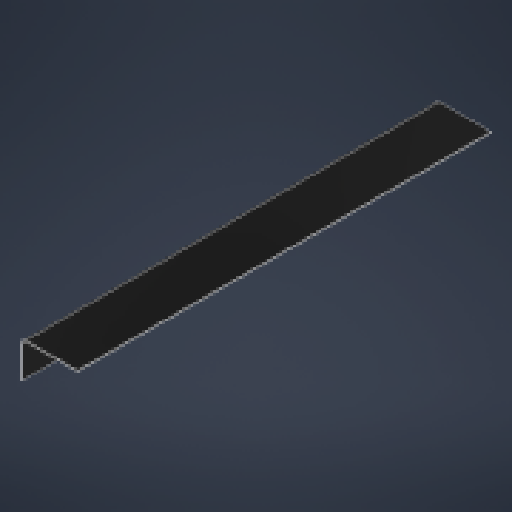
# Autodesk Inventor part: TopPlate
Saved by Autodesk Inventor 2023 (Build 270158000, 158)
## iProperties
Created: 2022-11-17
Part Number: TopPlate
Material: ABS Plastic
Document SubType Name: Modeling
Designer: kumpu
Density: 1.06 g/cm^3
Appearance: Smooth - Black
Mass: 160.66 g
Surface Area: 1935.06 cm^2
Volume: 151.566 cm^3
Author: kumpu
Autodesk Inventor part; units mm, degrees
ref_plane "YZ Plane" through (0, 0, 0) normal (1, 0, 0) x (0, 1, 0)
ref_plane "XZ Plane" through (0, 0, 0) normal (0, 1, 0) x (-1, 0, 0)
ref_plane "XY Plane" through (0, 0, 0) normal (0, 0, 1) x (1, 0, 0)
sketch "Sketch1" plane through (0, 0, 0) normal (0, 1, 0) x (-1, 0, 0)
  line L0 (41.275, 330.2) -> (-41.275, 330.2)
  line L1 (-41.275, 330.2) -> (-41.275, -330.2)
  line L2 (-41.275, -330.2) -> (41.275, -330.2)
  line L3 (41.275, -330.2) -> (41.275, 330.2)
  line L4 (41.275, 330.2) -> (-41.275, -330.2) construction
  line L5 (-41.275, 330.2) -> (41.275, -330.2) construction
  point P0 (0, 0)
  dimension "d0" = 82.55
  dimension "d1" = 660.4
  constraints: 12 end point, 2 midpoint, 2 parallel, 1 horizontal, 1 perpendicular
  measures "d0" distance of L2.end L1.end
  measures "d1" distance of L1.end L0.end
extrude "Extrusion1" add sketch "Sketch1" along normal mid plane 1.5875
sketch "Sketch2" plane through (41.275, 0.7937, -330.2) normal (0, 0, -1) x (-1, 0, 0)
  line L0 (90.4875, -7.9375) -> (90.4875, -58.7375)
  line L1 (90.4875, -58.7375) -> (88.9, -58.7375)
  line L2 (88.9, -58.7375) -> (88.9, -7.9375)
  arc A0 (88.9, -7.9375) -> (82.55, -1.5875) centre (82.55, -7.9375) ccw
  line L3 (82.55, -1.5875) -> (82.55, 0)
  arc A1 (90.4875, -7.9375) -> (82.55, 0) centre (82.55, -7.9375) ccw
  point P0 (41.275, -0.7937)
  dimension "d4" = 6.35
  dimension "d5" = 57.15
  dimension "d6" = 1.5875
  constraints: 8 end point, 4 point on circle, 2 centre point, 2 line through centre, 2 perpendicular, 2 tangent, 1 coincident, 1 concentric, 1 parallel, 1 point on line, 1 vertical
  measures "d4" radius of A0
  measures "d5" distance from line of L1 L3.start
  measures "d6" distance of L3.start L3.end
extrude "Extrusion2" add sketch "Sketch2" against normal blind 660.4
sketch "Sketch3" plane through (-49.2125, -57.9438, -330.2) normal (-1, 0, 0) x (0, 0, 1)
  arc A0 (518.9985, 0) -> (520.5697, 1.8143) centre (518.9985, 1.5875) ccw projected
  arc A1 (520.5697, 1.8143) -> (508, 12.7) centre (508, 0) ccw projected
  line L0 (497.2617, 12.7) -> (508, 12.7) projected
  line L1 (413.9219, 12.7) -> (497.2617, 12.7) projected
  line L2 (330.2, 12.7) -> (413.9219, 12.7) projected
  line L3 (226.8601, 12.7) -> (330.2, 12.7) projected
  line L4 (158.6559, 12.7) -> (226.8601, 12.7) projected
  line L5 (152.4, 12.7) -> (158.6559, 12.7) projected
  arc A2 (152.4, 12.7) -> (139.8303, 1.8143) centre (152.4, 0) ccw projected
  arc A3 (139.8303, 1.8143) -> (141.4015, 0) centre (141.4015, 1.5875) ccw projected
  line L6 (518.9985, 0) -> (141.4015, 0) projected
  line L7 (497.2617, 22.225) -> (508, 22.225)
  arc A4 (529.997, 3.175) -> (508, 22.225) centre (508, 0) ccw
  arc A5 (518.9985, -9.525) -> (529.997, 3.175) centre (518.9985, 1.5875) ccw
  line L8 (518.9985, -9.525) -> (141.4015, -9.525)
  arc A6 (130.403, 3.175) -> (141.4015, -9.525) centre (141.4015, 1.5875) ccw
  arc A7 (152.4, 22.225) -> (130.403, 3.175) centre (152.4, 0) ccw
  line L9 (152.4, 22.225) -> (158.6559, 22.225)
  line L10 (158.6559, 22.225) -> (226.8601, 22.225)
  line L11 (226.8601, 22.225) -> (330.2, 22.225)
  line L12 (330.2, 22.225) -> (413.9219, 22.225)
  line L13 (413.9219, 22.225) -> (497.2617, 22.225)
  point P0 (330.2, 57.9438)
  dimension "d9" = 9.525
  constraints: 14 end point, 8 point on circle, 4 centre point, 10 other
  measures "d9" distance between parallel lines of L1 L13
extrude "Extrusion3" cut sketch "Sketch3" against normal up to surface (1.5875 mm away) contours L6 A3 A2 L5 L4 L3 L2 L1 L0 A1 A0 | L7 A4 A5 L8 A6 A7 L9 L10 L11 L12 L13
sketch "Sketch5" plane through (-49.2125, -57.9438, -330.2) normal (-1, 0, 0) x (0, 0, 1)
  line L0 (515.6192, 11.1235) -> (519.405, 9.6946) projected
  line L1 (518.9828, 20.0348) -> (522.7587, 18.6096)
  line L2 (518.9828, 20.0348) -> (513.1799, 22.225)
  line L3 (513.1799, 22.225) -> (508, 22.225)
  arc A0 (529.997, 3.175) -> (508, 22.225) centre (508, 0) ccw projected
  line L4 (522.7587, 18.6096) -> (572.0643, 0)
  line L5 (529.997, 0) -> (660.4, 0) projected
  arc A1 (130.403, 3.175) -> (130.403, 0) centre (141.4015, 1.5875) ccw projected
  arc A2 (152.4, 22.225) -> (130.403, 3.175) centre (152.4, 0) ccw projected
  line L6 (152.4, 22.225) -> (508, 22.225) projected
  arc A3 (529.997, 3.175) -> (508, 22.225) centre (508, 0) ccw projected
  arc A4 (529.997, 0) -> (529.997, 3.175) centre (518.9985, 1.5875) ccw projected
  line L7 (529.997, 0) -> (660.4, 0) projected
  line L8 (660.4, 50.8) -> (660.4, 0) projected
  line L9 (0, 50.8) -> (660.4, 50.8) projected
  line L10 (0, 0) -> (0, 50.8) projected
  line L11 (0, 0) -> (130.403, 0) projected
  point P0 (330.2, 57.9438)
  dimension "d12" = 9.525
  constraints: 8 end point, 2 collinear, 1 horizontal, 1 parallel, 1 point on circle, 1 point on line, 1 tangent
  measures "d12" distance between parallel lines of L0 L1
extrude "Extrusion4" cut sketch "Sketch5" against normal up to surface (1.5875 mm away) contours L1 L4 L5 A4 A0 L3 L2
fillet "Fillet1" radius 3.175 2 edges at (-48.4188, -57.9438, -199.797) (-48.4188, -35.7187, 182.9799)
fillet "Fillet2" radius 3.175 4 edges at (-48.4188, -57.9438, -330.2) (41.275, 0, -330.2) (-48.4188, -57.9438, 330.2) (41.275, 0, 330.2)
body "Solid1"
